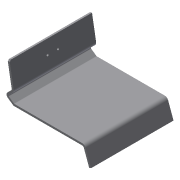
# Autodesk Inventor part: Ramp test
Saved by Autodesk Inventor 2015 SP1 (Build 190203100, 203)
## iProperties
Created: 2015-04-04
Part Number: Ramp test
Material: Generic
Document SubType Name: Sheet Metal
Designer: datenney
Density: 1 g/cm^3
Sheet Metal Rule: Default
Appearance: Default
Author: datenney
Autodesk Inventor part; units mm, degrees
ref_plane "YZ Plane" through (0, 0, 0) normal (1, 0, 0) x (0, 1, 0)
ref_plane "XZ Plane" through (0, 0, 0) normal (0, 1, 0) x (-1, 0, 0)
ref_plane "XY Plane" through (0, 0, 0) normal (0, 0, 1) x (1, 0, 0)
sketch "Sketch1" plane through (0, 0, 0) normal (0, 1, 0) x (-1, 0, 0)
  line L0 (98.933, -63.5) -> (-98.933, -63.5)
  line L1 (-98.933, -63.5) -> (-98.933, 63.5)
  line L2 (-98.933, 63.5) -> (98.933, 63.5)
  line L3 (98.933, 63.5) -> (98.933, -63.5)
  line L4 (98.933, -63.5) -> (-98.933, 63.5) construction
  line L5 (-98.933, -63.5) -> (98.933, 63.5) construction
  line L6 (-72.1614, -63.5) -> (-72.1614, 63.5)
  line L7 (60.833, 63.5) -> (60.833, -63.5)
  line L8 (48.133, -63.5) -> (48.133, 63.5)
  line L9 (35.433, -63.5) -> (35.433, 63.5)
  point P0 (0, 0)
  dimension "d0" = 197.866
  dimension "d1" = 127
  dimension "d2" = 38.1
  dimension "d3" = 26.7716
  dimension "d4" = 12.7
  dimension "d18" = 12.7
  constraints: 20 end point, 8 point on line, 4 vertical, 2 midpoint, 2 parallel, 1 horizontal, 1 perpendicular
  measures "d0" distance of L1.end L2.end
  measures "d1" distance of L0.end L1.end
  measures "d2" distance between parallel lines of L3 L7
  measures "d3" distance between parallel lines of L1 L6
  measures "d4" distance between parallel lines of L8 L7
  measures "d18" distance between parallel lines of L8 L9
extrude "Plate1" add sketch "Sketch1" along normal blind 3.048
fold "Fold1" angle 55 bend radius 2.54 thickness 3.048 k factor 0.44 line from (-60.833, 0, 63.5) to (-60.833, 0, -63.5) line at bend centre moving side (-1, 0, 0) folds toward (0, -1, 0)
fold "Fold2" angle 70 bend radius 2.54 thickness 3.048 k factor 0.44 line from (72.1614, 0, -63.5) to (72.1614, 0, 63.5) line at bend centre moving side (1, 0, 0) folds toward (0, -1, 0)
fold "Fold3" angle 100 bend radius 1.27 thickness 3.048 k factor 0.44 line from (-48.133, 0, -63.5) to (-48.133, 0, 63.5) line at bend centre moving side (-1, 0, 0) folds toward (0, 1, 0)
fold "Fold4" angle 35 bend radius 1.27 thickness 3.048 k factor 0.44 line from (-35.433, 0, -63.5) to (-35.433, 0, 63.5) line at bend centre moving side (-1, 0, 0) folds toward (0, 1, 0)
sketch "Sketch2" plane through (-45.1075, 56.8669, -63.5) normal (-0.9848078, -0.1736482, 0) x (0, 0, 1)
  line L0 (127, 0) -> (127, -19.05) construction
  line L1 (127, -36.2372) -> (127, 0) construction
  line L2 (127, -19.05) -> (71.501, -19.05) construction
  point P0 (63.5, -63.8358)
  point P1 (55.499, -19.05)
  dimension "d31" = 19.05
  dimension "d32" = 55.499
  dimension "d33" = 16.002
  constraints: 4 end point, 1 coincident, 1 horizontal, 1 horizontal alignment, 1 point on line
  measures "d31" distance of L0.start L0.end
  measures "d32" distance of L0.end L2.end
  measures "d33" distance of point (71.501, -19.05) point (55.499, -19.05)
hole "Hole1" at (-45.1075, 56.8669, 63.5) at (-41.7995, 38.1063, 8.001) at (-41.7995, 38.1063, -8.001) direction (0.9848078, 0.1736482, 0) diameter 3.175 end through all
equation "\"d18\" = d4"
equation "\"d6\" = BendReliefWidth"
equation "\"d7\" = BendReliefDepth"
equation "\"d8\" = MinimumRemnant"
equation "\"d9\" = BendRadius"
equation "\"d12\" = BendReliefWidth"
equation "\"d13\" = BendReliefDepth"
equation "\"d14\" = MinimumRemnant"
equation "\"d15\" = BendRadius"
equation "\"d19\" = BendReliefWidth"
equation "\"d20\" = BendReliefDepth"
equation "\"d21\" = MinimumRemnant"
equation "\"d22\" = BendRadius"
equation "\"d25\" = BendReliefWidth"
equation "\"d26\" = BendReliefDepth"
equation "\"d27\" = MinimumRemnant"
equation "\"d28\" = BendRadius"
equation "\"d39\" = Thickness"
equation "\"BendRadius\" = Thickness"
equation "\"BendReliefWidth\" = Thickness"
equation "\"BendReliefDepth\" = 0.5 * Thickness"
equation "\"CornerReliefSize\" = 4 * Thickness"
equation "\"MinimumRemnant\" = 2 * Thickness"
equation "\"TransitionRadius\" = BendRadius"
equation "\"JacobiRadiusSize\" = BendRadius"
equation "\"GapSize\" = Thickness"
equation "\"d5\" = BendRadius"
equation "\"Thickness\" = 3.048"
body "Solid1"
